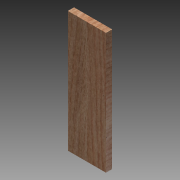
# Autodesk Inventor part: CNC-Z-axis - backplate
Saved by Autodesk Inventor 2015 (Build 190159000, 159)
## iProperties
Created: 2015-03-21
Part Number: CNC-Z-axis - backplate
Material: Generic
Document SubType Name: Modeling
Designer: Bangladesh
Density: 1 g/cm^3
Appearance: Default
Author: Bangladesh
Autodesk Inventor part; units mm, degrees
ref_plane "YZ Plane" through (0, 0, 0) normal (1, 0, 0) x (0, 1, 0)
ref_plane "XZ Plane" through (0, 0, 0) normal (0, 1, 0) x (-1, 0, 0)
ref_plane "XY Plane" through (0, 0, 0) normal (0, 0, 1) x (1, 0, 0)
sketch "Sketch2" plane through (0, 0, 0) normal (0, 0, 1) x (1, 0, 0)
  line L0 (-40, 127) -> (40, 127)
  line L1 (40, 127) -> (40, -127)
  line L2 (40, -127) -> (-40, -127)
  line L3 (-40, -127) -> (-40, 127)
  line L4 (-40, 127) -> (40, -127) construction
  line L5 (40, 127) -> (-40, -127) construction
  point P0 (0, 0)
  dimension "d1" = 80
  dimension "d2" = 254
  constraints: 12 end point, 2 midpoint, 2 parallel, 1 horizontal, 1 perpendicular
  measures "d1" distance of L1.end L2.end
  measures "d2" distance of L0.end L1.end
extrude "Extrusion1" add sketch "Sketch2" along normal mid plane 13
body "Solid1"
